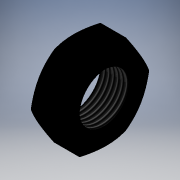
# Autodesk Inventor part: NT-05(63)_CE2
Saved by Autodesk Inventor 2017.3 (Build 213256000, 256)
## iProperties
Part Number: NT-05(63)_CE2
Material: Generic
Catalog Web Link: www.cadenas.de
Description: NT CE2-Rod End Nut
Vendor: SMC
Document SubType Name: Modeling
Designer: partserver
Manufacturer: SMC
Mass: 4.55003 g
Surface Area: 23.2976 cm^2
Volume: 4.55003 cm^3
Density: 1 g/cm^3
Appearance: PSOLRGB-0-0-0
Category: PARTsolutions
Company: SMC
Title: NT-05
Author: Cadenas PARTsolutions
Comments: Rod End Nut
PSOL_IDENT_0: {$CADENAS_DATA\23d-libs\smc_jp\actuator\stroke_reading_cylinders\ce2\accessories\ce2_nut.prj},159 {V
PSOL_IDENT_1: TYP=3D},{NB=NT-05(63)_CE2},{LINA=NT-05},{NN=NT CE2},{DATE=05.07.2021 01:49:15},{GEOMDATE=29.04.2019
PSOL_IDENT_2: 04:12:01},{VERSION=},{LINEID=110},{WBVAR=},{WBNUMERIC=}  {NB=NT-05(63)_CE2},{LINA=NT-05},{KT=DUMMY},
PSOL_IDENT_3: {PARTNO=NT-05},{BORE=63},{D=M18x1.5},{H=11},{B=27},{C=31.2},{DD=26},{DA=18.000},{DP=1.500},{MODEL=NT
PSOL_IDENT_4: -05}
NB: NT-05(63)_CE2
NN: NT CE2
NT: Rod End Nut
NBSYN: $PARTNO.($BORE.)_CE2
LINA: NT-05
CATALOG: SMC (JP
PARTNO: NT-05
BORE: 63
D: M18x1.5
H: 11
B: 27
C: 31.2
SUPPLIER: SMC
ARTICLENO: NT-05(63)_CE2
BOMINFO: NT-05
CREATOR: CADENAS GmbH
Autodesk Inventor part; units mm, degrees
sketch "Sketch_1" plane through (0, 0, 0) normal (0, 0, 1) x (1, 0, 0)
  line L0 (5.5, 0) -> (-5.5, 0)
  line L1 (-5.5, 13.5) -> (-5.5, 9)
  line L2 (-5.5, 9) -> (-4.688, 8.188)
  line L3 (-4.688, 8.188) -> (4.688, 8.188)
  line L4 (4.688, 8.188) -> (5.5, 9)
  line L5 (5.5, 9) -> (5.5, 13.5)
  line L6 (5.5, 13.5) -> (3.7102, 16.6)
  line L7 (3.7102, 16.6) -> (-3.7102, 16.6)
  line L8 (-3.7102, 16.6) -> (-5.5, 13.5)
  constraints: 18 end point
revolve "Revolution1" add sketch "Sketch_1" angle 360 about axis through (5.5, 0, 0) along (1, 0, 0)
thread "Thread1" size "M18x1.5" class "6H" standard "ISO Metric profile" full length
sketch "Sketch_2" plane through (0, 0, 0) normal (1, 0, 0) x (0, 1, 0)
  circle A0 centre (0, 0) radius 50
  line L0 (-7.7942, 13.5) -> (-15.5885, 0)
  line L1 (-15.5885, 0) -> (-7.7942, -13.5)
  line L2 (-7.7942, -13.5) -> (7.7942, -13.5)
  line L3 (7.7942, -13.5) -> (15.5885, 0)
  line L4 (15.5885, 0) -> (7.7942, 13.5)
  line L5 (7.7942, 13.5) -> (-7.7942, 13.5)
  constraints: 12 end point, 1 centre point
extrude "Extrusion1" cut sketch "Sketch_2" along normal mid plane 22
ref_plane "B1_XY" through (5.5, 0, 13.5) normal (1, 0, 0) x (0, 0, -1)
ref_plane "B1_YZ" through (5.5, 0, 13.5) normal (0, 0, -1) x (0, 1, 0)
ref_plane "B1_ZX" through (5.5, 0, 13.5) normal (0, 1, 0) x (1, 0, 0)
ref_plane "N_R_XY" through (0, 0, 0) normal (1, 0, 0) x (0, 0, -1)
ref_plane "N_R_YZ" through (0, 0, 0) normal (0, 0, -1) x (0, 1, 0)
ref_plane "N_R_ZX" through (0, 0, 0) normal (0, 1, 0) x (1, 0, 0)
body "Solid1"
